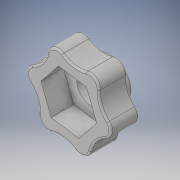
# Autodesk Inventor part: BackNut
Saved by Autodesk Inventor 2016 (Build 200138000, 138)
## iProperties
Created: 2017-03-07
Part Number: BackNut
Material: Generic
Document SubType Name: Modeling
Designer: peter
Density: 1 g/cm^3
Appearance: Default
Mass: 1.34669 g
Surface Area: 12.3665 cm^2
Volume: 1.34669 cm^3
Author: peter
Autodesk Inventor part; units mm, degrees
ref_plane "YZ Plane" through (0, 0, 0) normal (1, 0, 0) x (0, 1, 0)
ref_plane "XZ Plane" through (0, 0, 0) normal (0, 1, 0) x (-1, 0, 0)
ref_plane "XY Plane" through (0, 0, 0) normal (0, 0, 1) x (1, 0, 0)
sketch "Sketch1" plane through (0, 0, 0) normal (1, 0, 0) x (0, 1, 0)
  line L0 (0, 0) -> (0, 9.586) construction
  line L1 (3.302, 0) -> (4.3656, 0)
  line L2 (4.7625, 0.3969) -> (4.7625, 3.175)
  line L3 (4.7625, 3.175) -> (3.302, 3.175)
  line L4 (3.302, 3.175) -> (3.302, 0)
  line L5 (3.302, 3.175) -> (9.525, 3.175)
  line L6 (9.525, 3.175) -> (9.525, 9.1281)
  line L7 (9.1281, 9.525) -> (3.302, 9.525)
  line L8 (3.302, 9.525) -> (3.302, 3.175)
  arc A0 (4.3656, 0) -> (4.7625, 0.3969) centre (4.3656, 0.3969) ccw
  arc A1 (9.525, 9.1281) -> (9.1281, 9.525) centre (9.1281, 9.1281) ccw
  line L9 (9.1281, 9.525) -> (9.525, 9.525)
  line L10 (9.525, 9.1281) -> (9.525, 9.525)
  point P0 (4.7625, 0)
  point P1 (9.525, 3.175)
  point P2 (9.525, 3.175)
  dimension "d7" = 0
  dimension "d0" = 3.175
  dimension "d1" = 3.302
  dimension "d4" = 6.35
  dimension "d5" = 9.525
  dimension "d6" = 0.3969
  dimension "d11" = 4.7625
  constraints: 22 end point, 6 point on line, 4 horizontal, 4 parallel, 4 point on circle, 4 tangent, 3 vertical, 2 centre point, 2 perpendicular, 1 equal radius, 4 other
  measures "d0" distance of point (4.763, 0) L2.end
  measures "d1" distance between parallel lines of L0 L4
  measures "d4" distance of point (9.525, 3.175) L9.end
  measures "d5" distance between parallel lines of L0 L6
  measures "d6" radius of A0
  measures "d11" distance between parallel lines of L0 L2
revolve "Revolution1" add sketch "Sketch1" angle 360 about axis through (0, 0, 0) along (0, 0, 1)
sketch "Sketch2" plane through (0, 0, 9.525) normal (0, 0, 1) x (1, 0, 0)
  line L0 (2.3274, -5.9081) -> (-3.9528, -4.9697)
  line L1 (-3.9528, -4.9697) -> (-6.2803, 0.9384)
  line L2 (-6.2803, 0.9384) -> (-2.3274, 5.9081)
  line L3 (-2.3274, 5.9081) -> (3.9528, 4.9697)
  line L4 (3.9528, 4.9697) -> (6.2803, -0.9384)
  line L5 (6.2803, -0.9384) -> (2.3274, -5.9081)
  point P0 (0, 0)
  point P1 (0, 0)
  dimension "d9" = 12.7
  dimension "d10" = 10.9985
  constraints: 12 end point, 1 coincident, 13 other
  measures "d9" distance of L0.end L3.end
  measures "d10" distance between parallel lines of L0 L3
extrude "Extrusion1" cut sketch "Sketch2" against normal blind 5.08
sketch "Sketch3" plane through (0, 0, 9.525) normal (0, 0, 1) x (1, 0, 0)
  line L0 (6.2803, -0.9384) -> (2.3274, -5.9081) projected
  line L1 (2.3274, -5.9081) -> (-3.9528, -4.9697) projected
  line L2 (-3.9528, -4.9697) -> (-6.2803, 0.9384) projected
  line L3 (-6.2803, 0.9384) -> (-2.3274, 5.9081) projected
  line L4 (-2.3274, 5.9081) -> (3.9528, 4.9697) construction
  line L5 (3.9528, 4.9697) -> (6.2803, -0.9384) projected
  circle A0 centre (0, 0) radius 9.525 construction
  line L6 (0, 0) -> (-3.4911, 8.8621) construction
  line L7 (0, 0) -> (5.9293, 7.4545) construction
  line L8 (0, 0) -> (1.4076, 9.4204) construction
  arc A1 (-1.4653, 8.6464) -> (-3.4911, 8.8621) centre (-2.6847, 6.8151) ccw
  arc A2 (5.9293, 7.4545) -> (3.9289, 7.8404) centre (4.5597, 5.7326) ccw
  arc A3 (-1.4653, 8.6464) -> (3.9289, 7.8404) centre (2.0898, 13.9856) ccw
  arc A4 (5.9293, 7.4545) -> (-3.4911, 8.8621) centre (0, 0) ccw
  circle A5 centre (0, 0) radius 9.525 construction
  dimension "d14" = 30
  constraints: 11 point on circle, 6 end point, 5 point on line, 4 centre point, 2 coincident, 2 tangent, 2 other
  measures "d14" angle of L7 L8
extrude "Extrusion2" cut sketch "Sketch3" against normal through all
pattern_circular "Circular Pattern1" count 6 over 360 about axis through (0, 0, -10) along (0, 0, 1) of "Extrusion2"
fillet "Fillet1" radius 0.4064 24 edges at (-3.4911, 8.8621, 9.525) (-6.0469, 4.8096, 9.525) (-9.4204, 1.4076, 9.525) (-7.1887, -2.8319, 9.525) (-5.9293, -7.4545, 9.525) (-1.1418, -7.6415, 9.525) (3.4911, -8.8621, 9.525) (6.0469, -4.8096, 9.525) (9.4204, -1.4076, 9.525) (7.1887, 2.8319, 9.525) (5.9293, 7.4545, 9.525) (1.1418, 7.6415, 9.525) (5.9293, 7.4545, 3.175) (7.1887, 2.8319, 3.175) (9.4204, -1.4076, 3.175) (6.0469, -4.8096, 3.175) (3.4911, -8.8621, 3.175) (-1.1418, -7.6415, 3.175) (-5.9293, -7.4545, 3.175) (-7.1887, -2.8319, 3.175) (-9.4204, 1.4076, 3.175) (-6.0469, 4.8096, 3.175) (-3.4911, 8.8621, 3.175) (1.1418, 7.6415, 3.175)
body "Solid1"
